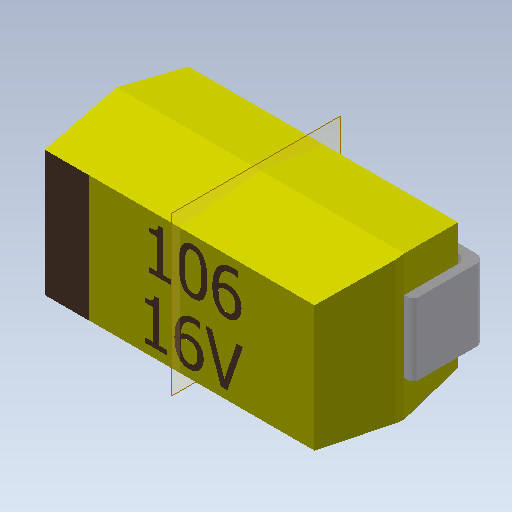
# Autodesk Inventor part: tantalum 10uF
Saved by Autodesk Inventor 2020.3 (Build 243373000, 373)
## iProperties
Created: 2015-04-13
Part Number: tantalum 10uF
Material: Generic
Document SubType Name: Modeling
Designer: s42851
Density: 1 g/cm^3
Appearance: Metal 2400F Hot
Author: s42851
Autodesk Inventor part; units mm, degrees
ref_plane "XZ Plane" through (0, 0, 0) normal (0, 1, 0) x (-1, 0, 0)
ref_plane "XY Plane" through (0, 0, 0) normal (0, 0, 1) x (1, 0, 0)
sketch "Sketch1" plane through (0, 0, 0) normal (0, 0, 1) x (1, 0, 0)
  line L0 (0, 0) -> (3.2, 0)
  line L1 (3.2, 0) -> (3.2, 1.6)
  line L2 (3.2, 1.6) -> (0, 1.6)
  line L3 (0, 1.6) -> (0, 0)
  dimension "d0" = 1.6
  dimension "d1" = 3.2
  constraints: 8 end point, 2 parallel, 1 horizontal, 1 perpendicular
  measures "d0" distance of L2.end L0.start
  measures "d1" distance of L0.start L0.end
extrude "Extrusion1" add sketch "Sketch1" along normal blind 1.6
chamfer "Chamfer2" distance 0.9 distance2 0.1 1 edges at (1.6, 0, 1.6) measured on face at (1.0667, 0, 0.5333)
chamfer "Chamfer3" distance 0.9 distance2 0.1 1 edges at (1.6, 1.6, 1.6) measured on face at (2.1333, 1.6, 0.5333)
chamfer "Chamfer4" distance 0.9 distance2 0.1 1 edges at (0, 0.8, 1.6) measured on face at (0, 1.0333, 1)
chamfer "Chamfer5" distance 0.7 distance2 0.1 1 edges at (1.6, 0, 0) measured on face at (1.0667, 0, 0.2333)
chamfer "Chamfer6" distance 0.7 distance2 0.1 1 edges at (1.6, 1.6, 0) measured on face at (2.1333, 1.6, 0.2333)
chamfer "Chamfer7" distance 0.7 distance2 0.1 1 edges at (0, 0.8, 0) measured on face at (0, 0.5665, 0.4663)
chamfer "Chamfer8" distance 0.7 distance2 0.1 1 edges at (3.2, 0.8, 0) measured on face at (3.2, 0.5667, 1)
sketch "Sketch2" plane through (0, 0, 0) normal (1, 0, 0) x (0, 1, 0)
  line L0 (0.1, 0) -> (0, 0.7) projected
  line L1 (1.6, 0.7) -> (0, 0.7) projected
  line L2 (1.6, 0.7) -> (1.5, 0) projected
  line L3 (1.5, 0) -> (0.1, 0) projected
  line L4 (1.2, 0.7) -> (0.4, 0.7)
  line L5 (0.4, 0.7) -> (0.4, -0.1)
  line L6 (0.4, -0.1) -> (1.2, -0.1)
  line L7 (1.2, -0.1) -> (1.2, 0.7)
  point P0 (0, 0)
  dimension "d28" = 0.8
  dimension "d29" = 0.4
  dimension "d30" = 0.1
  constraints: 8 end point, 2 parallel, 1 horizontal, 1 perpendicular, 1 point on line
  measures "d28" distance of L4.start L4.end
  measures "d29" distance from line of L0.end L5
  measures "d30" distance between parallel lines of L3 L6
extrude "Extrusion2" add sketch "Sketch2" against normal blind 0.1 contours L5 L1 L7 L3 | L3 L7 L6 L5
sketch "Sketch3" plane through (0, 0, 0) normal (1, 0, 0) x (0, 0, -1)
  line L0 (-0.7, 0.4) -> (0.1, 0.4) projected
  line L1 (0.1, 1.2) -> (0, 1.2)
  line L2 (0, 1.2) -> (0, 0.4)
  line L3 (0, 0.4) -> (0.1, 0.4)
  line L4 (0.1, 0.4) -> (0.1, 1.2)
  point P0 (0, 0)
  dimension "d33" = 0.1
  constraints: 8 end point, 2 parallel, 1 horizontal, 1 perpendicular, 1 point on line
  measures "d33" distance between parallel lines of L4 L2
extrude "Extrusion3" add sketch "Sketch3" along normal blind 0.8
ref_plane "Work Plane1" through (1.6, 0, 0) normal (1, 0, 0) x (0, 1, 0)
mirror "Mirror1" about plane through (1.6, 0, 0) normal (1, 0, 0) of "Extrusion2", "Extrusion3"
fillet "Fillet1" radius 0.05 2 edges at (3.3, 0.8, 0.7) (-0.1, 0.8, 0.7)
fillet "Fillet2" radius 0.1 4 edges at (3.3, 0.8, -0.1) (3.2, 0.8, 0) (-0.1, 0.8, -0.1) (0, 0.8, 0)
chamfer "Chamfer9" distance 0.8 distance2 0.1 1 edges at (3.2, 0.8, 1.6) measured on face at (3.2, 0.9333, 1.3)
sketch "Sketch4" plane through (0, 0, 1.6) normal (0, 0, 1) x (1, 0, 0)
  line L0 (3.1, 0.1) -> (0.1, 0.1) projected
  line L1 (0.1, 1.5) -> (0.5939, 1.5)
  line L2 (0.5939, 1.5) -> (0.5939, 0.1)
  line L3 (0.5939, 0.1) -> (0.1, 0.1)
  line L4 (0.1, 0.1) -> (0.1, 1.5)
  point P0 (0, 0)
  constraints: 8 end point, 2 parallel, 1 horizontal, 1 perpendicular, 1 point on line
extrude "Extrusion4" add sketch "Sketch4" along normal blind 0.001
sketch "Sketch5" plane through (0, 0, 1.6) normal (0, 0, 1) x (1, 0, 0)
  line L0 (1.1862, 1.409) -> (2.532, 1.409) construction
  line L1 (2.532, 1.409) -> (2.532, 0.7466) construction
  line L2 (2.532, 0.7466) -> (1.1862, 0.7466) construction
  line L3 (1.1862, 0.7466) -> (1.1862, 1.409) construction
  line L4 (1.1402, 0.7075) -> (2.486, 0.7075) construction
  line L5 (2.486, 0.7075) -> (2.486, 0.0451) construction
  line L6 (2.486, 0.0451) -> (1.1402, 0.0451) construction
  line L7 (1.1402, 0.0451) -> (1.1402, 0.7075) construction
  line L8 (1.5059, 0.8989) -> (1.262, 0.8989)
  line L9 (1.262, 0.8989) -> (1.262, 0.9499)
  line L10 (1.262, 0.9499) -> (1.3527, 0.9499)
  line L11 (1.3527, 0.9499) -> (1.3527, 1.285)
  line L12 (1.3527, 1.285) -> (1.262, 1.285)
  line L13 (1.262, 1.285) -> (1.262, 1.3308)
  spline S0 degree 2 poles (1.262, 1.3308) (1.3134, 1.3308) (1.362, 1.36) (1.3653, 1.4005) knots 0 0 0 1 2 2 2
  line L14 (1.3653, 1.4005) -> (1.4172, 1.4005)
  line L15 (1.4172, 1.4005) -> (1.4172, 0.9499)
  line L16 (1.4172, 0.9499) -> (1.5059, 0.9499)
  line L17 (1.5059, 0.9499) -> (1.5059, 0.8989)
  spline S1 degree 2 poles (1.909, 1.1489) (1.909, 1.0144) (1.8308, 0.8884) (1.7494, 0.8884) knots 0 0 0 1 2 2 2
  spline S2 degree 2 poles (1.7494, 0.8884) (1.6667, 0.8884) (1.5894, 1.0168) (1.5894, 1.1485) knots 0 0 0 1 2 2 2
  spline S3 degree 2 poles (1.5894, 1.1485) (1.5894, 1.2838) (1.6676, 1.409) (1.7494, 1.409) knots 0 0 0 1 2 2 2
  spline S4 degree 2 poles (1.7494, 1.409) (1.8317, 1.409) (1.909, 1.2794) (1.909, 1.1489) knots 0 0 0 1 2 2 2
  spline S5 degree 2 poles (1.8231, 0.9965) (1.8329, 1.0213) (1.841, 1.0974) (1.841, 1.1489) knots 0 0 0 1 2 2 2
  spline S6 degree 2 poles (1.841, 1.1489) (1.841, 1.2003) (1.8329, 1.2761) (1.8227, 1.3016) knots 0 0 0 1 2 2 2
  spline S7 degree 2 poles (1.8227, 1.3016) (1.8126, 1.3272) (1.7774, 1.3535) (1.7494, 1.3535) knots 0 0 0 1 2 2 2
  spline S8 degree 2 poles (1.7494, 1.3535) (1.7214, 1.3535) (1.6854, 1.3272) (1.6749, 1.3008) knots 0 0 0 1 2 2 2
  spline S9 degree 2 poles (1.6749, 1.3008) (1.6647, 1.2753) (1.6574, 1.1975) (1.6574, 1.1485) knots 0 0 0 1 2 2 2
  spline S10 degree 2 poles (1.6574, 1.1485) (1.6574, 1.0958) (1.6639, 1.0253) (1.6744, 0.9978) knots 0 0 0 1 2 2 2
  spline S11 degree 2 poles (1.6744, 0.9978) (1.6842, 0.9718) (1.7202, 0.9439) (1.7494, 0.9439) knots 0 0 0 1 2 2 2
  spline S12 degree 2 poles (1.7494, 0.9439) (1.777, 0.9439) (1.813, 0.9702) (1.8231, 0.9965) knots 0 0 0 1 2 2 2
  spline S13 degree 2 poles (2.2891, 1.061) (2.2891, 1.0225) (2.2636, 0.9572) (2.2421, 0.9354) knots 0 0 0 1 2 2 2
  spline S14 degree 2 poles (2.2421, 0.9354) (2.2198, 0.9123) (2.1639, 0.8884) (2.1303, 0.8884) knots 0 0 0 1 2 2 2
  spline S15 degree 2 poles (2.1303, 0.8884) (2.0966, 0.8884) (2.0411, 0.911) (2.0201, 0.9337) knots 0 0 0 1 2 2 2
  spline S16 degree 2 poles (2.0201, 0.9337) (1.9941, 0.9609) (1.965, 1.052) (1.965, 1.1185) knots 0 0 0 1 2 2 2
  spline S17 degree 2 poles (1.965, 1.1185) (1.965, 1.1837) (1.9917, 1.2887) (2.0197, 1.3276) knots 0 0 0 1 2 2 2
  spline S18 degree 2 poles (2.0197, 1.3276) (2.0468, 1.3657) (2.1327, 1.4082) (2.189, 1.4082) knots 0 0 0 1 2 2 2
  spline S19 degree 2 poles (2.189, 1.4082) (2.2056, 1.4082) (2.2348, 1.405) (2.2458, 1.4013) knots 0 0 0 1 2 2 2
  line L18 (2.2458, 1.4013) -> (2.2458, 1.3369)
  line L19 (2.2458, 1.3369) -> (2.2429, 1.3369)
  spline S20 degree 2 poles (2.2429, 1.3369) (2.2336, 1.3418) (2.1996, 1.3503) (2.1801, 1.3503) knots 0 0 0 1 2 2 2
  spline S21 degree 2 poles (2.1801, 1.3503) (2.1177, 1.3503) (2.0411, 1.266) (2.0338, 1.1833) knots 0 0 0 1 2 2 2
  spline S22 degree 2 poles (2.0338, 1.1833) (2.0578, 1.1999) (2.108, 1.2182) (2.138, 1.2182) knots 0 0 0 1 2 2 2
  spline S23 degree 2 poles (2.138, 1.2182) (2.1672, 1.2182) (2.2109, 1.2064) (2.2348, 1.1886) knots 0 0 0 1 2 2 2
  spline S24 degree 2 poles (2.2348, 1.1886) (2.2624, 1.1679) (2.2891, 1.1039) (2.2891, 1.061) knots 0 0 0 1 2 2 2
  spline S25 degree 2 poles (2.221, 1.0581) (2.221, 1.0889) (2.2048, 1.1307) (2.187, 1.1452) knots 0 0 0 1 2 2 2
  spline S26 degree 2 poles (2.187, 1.1452) (2.1736, 1.1558) (2.1404, 1.1627) (2.123, 1.1627) knots 0 0 0 1 2 2 2
  spline S27 degree 2 poles (2.123, 1.1627) (2.0995, 1.1627) (2.0553, 1.1485) (2.0338, 1.1351) knots 0 0 0 1 2 2 2
  spline S28 degree 2 poles (2.0338, 1.1351) (2.0334, 1.1278) (2.0326, 1.114) (2.0326, 1.1035) knots 0 0 0 1 2 2 2
  spline S29 degree 2 poles (2.0326, 1.1035) (2.0326, 1.0516) (2.0529, 0.988) (2.0683, 0.9714) knots 0 0 0 1 2 2 2
  spline S30 degree 2 poles (2.0683, 0.9714) (2.0825, 0.9556) (2.1133, 0.9431) (2.1307, 0.9431) knots 0 0 0 1 2 2 2
  spline S31 degree 2 poles (2.1307, 0.9431) (2.1712, 0.9431) (2.221, 1.0006) (2.221, 1.0581) knots 0 0 0 1 2 2 2
  line L20 (1.4599, 0.1982) -> (1.216, 0.1982)
  line L21 (1.216, 0.1982) -> (1.216, 0.2493)
  line L22 (1.216, 0.2493) -> (1.3067, 0.2493)
  line L23 (1.3067, 0.2493) -> (1.3067, 0.5843)
  line L24 (1.3067, 0.5843) -> (1.216, 0.5843)
  line L25 (1.216, 0.5843) -> (1.216, 0.6301)
  spline S32 degree 2 poles (1.216, 0.6301) (1.2674, 0.6301) (1.316, 0.6593) (1.3193, 0.6998) knots 0 0 0 1 2 2 2
  line L26 (1.3193, 0.6998) -> (1.3712, 0.6998)
  line L27 (1.3712, 0.6998) -> (1.3712, 0.2493)
  line L28 (1.3712, 0.2493) -> (1.4599, 0.2493)
  line L29 (1.4599, 0.2493) -> (1.4599, 0.1982)
  spline S33 degree 2 poles (1.8679, 0.3603) (1.8679, 0.3218) (1.8424, 0.2566) (1.8209, 0.2347) knots 0 0 0 1 2 2 2
  spline S34 degree 2 poles (1.8209, 0.2347) (1.7986, 0.2116) (1.7427, 0.1877) (1.7091, 0.1877) knots 0 0 0 1 2 2 2
  spline S35 degree 2 poles (1.7091, 0.1877) (1.6754, 0.1877) (1.6199, 0.2104) (1.5989, 0.2331) knots 0 0 0 1 2 2 2
  spline S36 degree 2 poles (1.5989, 0.2331) (1.5729, 0.2602) (1.5438, 0.3514) (1.5438, 0.4178) knots 0 0 0 1 2 2 2
  spline S37 degree 2 poles (1.5438, 0.4178) (1.5438, 0.4831) (1.5705, 0.588) (1.5985, 0.6269) knots 0 0 0 1 2 2 2
  spline S38 degree 2 poles (1.5985, 0.6269) (1.6256, 0.665) (1.7115, 0.7075) (1.7678, 0.7075) knots 0 0 0 1 2 2 2
  spline S39 degree 2 poles (1.7678, 0.7075) (1.7844, 0.7075) (1.8136, 0.7043) (1.8246, 0.7006) knots 0 0 0 1 2 2 2
  line L30 (1.8246, 0.7006) -> (1.8246, 0.6362)
  line L31 (1.8246, 0.6362) -> (1.8217, 0.6362)
  spline S40 degree 2 poles (1.8217, 0.6362) (1.8124, 0.6411) (1.7784, 0.6496) (1.7589, 0.6496) knots 0 0 0 1 2 2 2
  spline S41 degree 2 poles (1.7589, 0.6496) (1.6965, 0.6496) (1.6199, 0.5653) (1.6126, 0.4826) knots 0 0 0 1 2 2 2
  spline S42 degree 2 poles (1.6126, 0.4826) (1.6366, 0.4993) (1.6868, 0.5175) (1.7168, 0.5175) knots 0 0 0 1 2 2 2
  spline S43 degree 2 poles (1.7168, 0.5175) (1.746, 0.5175) (1.7897, 0.5057) (1.8136, 0.4879) knots 0 0 0 1 2 2 2
  spline S44 degree 2 poles (1.8136, 0.4879) (1.8412, 0.4673) (1.8679, 0.4032) (1.8679, 0.3603) knots 0 0 0 1 2 2 2
  spline S45 degree 2 poles (1.7998, 0.3574) (1.7998, 0.3882) (1.7836, 0.43) (1.7658, 0.4446) knots 0 0 0 1 2 2 2
  spline S46 degree 2 poles (1.7658, 0.4446) (1.7524, 0.4551) (1.7192, 0.462) (1.7018, 0.462) knots 0 0 0 1 2 2 2
  spline S47 degree 2 poles (1.7018, 0.462) (1.6783, 0.462) (1.6341, 0.4478) (1.6126, 0.4344) knots 0 0 0 1 2 2 2
  spline S48 degree 2 poles (1.6126, 0.4344) (1.6122, 0.4271) (1.6114, 0.4134) (1.6114, 0.4028) knots 0 0 0 1 2 2 2
  spline S49 degree 2 poles (1.6114, 0.4028) (1.6114, 0.351) (1.6317, 0.2873) (1.6471, 0.2707) knots 0 0 0 1 2 2 2
  spline S50 degree 2 poles (1.6471, 0.2707) (1.6613, 0.2549) (1.6921, 0.2424) (1.7095, 0.2424) knots 0 0 0 1 2 2 2
  spline S51 degree 2 poles (1.7095, 0.2424) (1.75, 0.2424) (1.7998, 0.2999) (1.7998, 0.3574) knots 0 0 0 1 2 2 2
  line L32 (2.3039, 0.6982) -> (2.1317, 0.1982)
  line L33 (2.1317, 0.1982) -> (2.06, 0.1982)
  line L34 (2.06, 0.1982) -> (1.8878, 0.6982)
  line L35 (1.8878, 0.6982) -> (1.9591, 0.6982)
  line L36 (1.9591, 0.6982) -> (2.0977, 0.2829)
  line L37 (2.0977, 0.2829) -> (2.2362, 0.6982)
  line L38 (2.2362, 0.6982) -> (2.3039, 0.6982)
  point P0 (0, 0)
  constraints: 4 other
extrude "Extrusion5" add sketch "Sketch5" along normal blind 0.001
body "Solid1"
